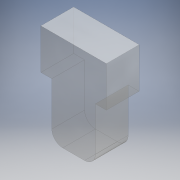
# Autodesk Inventor part: BBGW Case Button
Saved by Autodesk Inventor 2016 (Build 200138000, 138)
## iProperties
Created: 2016-06-26
Part Number: BBGW Case Button
Material: Acrylic, Clear
Document SubType Name: Modeling
Designer: Jacob
Density: 1.19 g/cm^3
Appearance: Transparent - Clear
Author: Jacob
Autodesk Inventor part; units mm, degrees
ref_plane "YZ Plane" through (0, 0, 0) normal (1, 0, 0) x (0, 1, 0)
ref_plane "XZ Plane" through (0, 0, 0) normal (0, 1, 0) x (-1, 0, 0)
ref_plane "XY Plane" through (0, 0, 0) normal (0, 0, 1) x (1, 0, 0)
sketch "Sketch1" plane through (0, 0, 0) normal (0, 1, 0) x (-1, 0, 0)
  line L0 (0, 0) -> (6, 0)
  line L1 (6, 0) -> (6, -3.7)
  line L2 (6, -3.7) -> (5, -3.7)
  line L3 (5, -3.7) -> (5, -8.7)
  line L4 (5, -8.7) -> (1, -8.7)
  line L5 (1, -8.7) -> (1, -3.7)
  line L6 (1, -3.7) -> (0, -3.7)
  line L7 (0, -3.7) -> (0, 0)
  dimension "d0" = 6
  dimension "d1" = 3.7
  dimension "d2" = 1
  dimension "d3" = 5
  dimension "d4" = 4
  dimension "d5" = 5
  dimension "d6" = 1
  constraints: 16 end point, 4 perpendicular, 2 point on line, 1 horizontal
  measures "d0" distance of L0.start L0.end
  measures "d1" distance of L0.end L1.end
  measures "d2" distance of L1.end L2.end
  measures "d3" distance of L2.end L3.end
  measures "d4" distance of L3.end L4.end
  measures "d5" distance of L4.end L5.end
  measures "d6" distance of L5.end L6.end
extrude "Extrusion1" add sketch "Sketch1" along normal blind 3
fillet "Fillet1" radius 1 2 edges at (-1, 1.5, -8.7) (-5, 1.5, -8.7)
body "Solid1"
